Autodesk Fusion 360 part; units mm, degrees
note: some values were not read from the file. Set by a fixed rule: which sketch regions a step uses.
(part 5 of 7)
  line L178 (-125, 205) -> (-105, 195)
  line L179 (-36.1991, -37.2933) -> (-30, -37.2933)
  line L180 (-60.0369, -43.8903) -> (-55.0369, -43.8903)
  line L181 (-55.0369, -43.8903) -> (-55.0369, -37.2933)
  line L182 (-55.0369, -37.2933) -> (-60, -37.2933)
  line L183 (-60, -37.2933) -> (-60, 10)
  line L184 (-60, 10) -> (-55, 10)
  constraint vertical L132
  constraint parallel L131 L133
  constraint parallel L132 L134
  constraint parallel L134 L135
  constraint parallel L134 L137
  constraint parallel L136 L138
  constraint parallel L133 L139
  constraint vertical L140
  constraint parallel L133 L141
  constraint parallel L140 L142
  constraint parallel L142 L143
  constraint parallel L143 L145
  constraint parallel L144 L146
  constraint parallel L139 L147
  constraint parallel L143 L148
  constraint parallel L139 L149
  constraint parallel L143 L150
  constraint parallel L143 L151
  constraint parallel L146 L152
  constraint parallel L151 L153
  constraint parallel L152 L154
  constraint parallel L147 L155
  constraint parallel L151 L156
  constraint parallel L147 L157
  constraint parallel L151 L158
  constraint parallel L151 L159
  constraint parallel L152 L160
  constraint parallel L151 L161
  constraint parallel L160 L162
  constraint parallel L155 L163
  constraint parallel L159 L164
  constraint parallel L163 L165
  constraint parallel L159 L166
  constraint parallel L159 L167
  constraint parallel L159 L169
  constraint parallel L168 L170
  constraint parallel L163 L171
  constraint parallel L167 L172
  constraint parallel L171 L173
  constraint parallel L167 L174
  constraint vertical L175
  constraint parallel L175 L177
  constraint parallel L176 L178
sketch "Sketch89" plane through (0, 116.2145, -31.1396) normal (0, 0.965926, -0.258819) x (-1, 0, 0)
  line L0 (-80, 205) -> (-100, 195)
  line L1 (-100, 195) -> (-100, 200)
  line L2 (-100, 200) -> (-80, 210)
  line L3 (-80, 210) -> (-80, 205)
  line L4 (-105, 170) -> (-105, 165)
  line L5 (-105, 165) -> (-125, 175)
  line L6 (-125, 175) -> (-125, 180)
  line L7 (-125, 180) -> (-105, 170)
  line L8 (-80, 165) -> (-100, 155)
  line L9 (-100, 155) -> (-100, 160)
  line L10 (-100, 160) -> (-80, 170)
  line L11 (-80, 170) -> (-80, 165)
  line L12 (-80, 155) -> (-100, 145)
  line L13 (-100, 145) -> (-100, 150)
  line L14 (-100, 150) -> (-80, 160)
  line L15 (-80, 160) -> (-80, 155)
  line L16 (-105, 180) -> (-105, 175)
  line L17 (-105, 175) -> (-125, 185)
  line L18 (-125, 185) -> (-125, 190)
  line L19 (-125, 190) -> (-105, 180)
  line L20 (-80, 195) -> (-100, 185)
  line L21 (-100, 185) -> (-100, 190)
  line L22 (-100, 190) -> (-80, 200)
  line L23 (-80, 200) -> (-80, 195)
  line L24 (-105, 200) -> (-105, 195)
  line L25 (-105, 195) -> (-125, 205)
  line L26 (-125, 205) -> (-125, 210)
  line L27 (-125, 210) -> (-105, 200)
  line L28 (-105, 160) -> (-105, 155)
  line L29 (-105, 155) -> (-125, 165)
  line L30 (-125, 165) -> (-125, 170)
  line L31 (-125, 170) -> (-105, 160)
  line L32 (-80, 175) -> (-100, 165)
  line L33 (-100, 165) -> (-100, 170)
  line L34 (-100, 170) -> (-80, 180)
  line L35 (-80, 180) -> (-80, 175)
  line L36 (-105, 150) -> (-105, 145)
  line L37 (-105, 145) -> (-125, 155)
  line L38 (-125, 155) -> (-125, 160)
  line L39 (-125, 160) -> (-105, 150)
  line L40 (-105, 190) -> (-105, 185)
  line L41 (-105, 185) -> (-125, 195)
  line L42 (-125, 195) -> (-125, 200)
  line L43 (-125, 200) -> (-105, 190)
  line L44 (-80, 185) -> (-100, 175)
  line L45 (-100, 175) -> (-100, 180)
  line L46 (-100, 180) -> (-80, 190)
  line L47 (-80, 190) -> (-80, 185)
  line L48 (-35.9419, 179.9959) -> (-35.9419, 150.9959)
  line L49 (-35.9419, 150.9959) -> (-72.9419, 150.9959)
  line L50 (-72.9419, 150.9959) -> (-72.9419, 179.9959)
  line L51 (-72.9419, 179.9959) -> (-35.9419, 179.9959)
  line L52 (25, 155) -> (0, 145)
  line L53 (0, 145) -> (0, 150)
  line L54 (0, 150) -> (25, 160)
  line L55 (25, 160) -> (25, 155)
  line L56 (25, 195) -> (0, 185)
  line L57 (0, 185) -> (0, 190)
  line L58 (0, 190) -> (25, 200)
  line L59 (25, 200) -> (25, 195)
  line L60 (-30, 180) -> (-30, 184.9041)
  line L61 (-30, 184.9041) -> (-5, 180)
  line L62 (-5, 180) -> (-5, 175)
  line L63 (-5, 175) -> (-30, 180)
  line L64 (-30, 150) -> (-30, 155)
  line L65 (-30, 155) -> (-5, 150)
  line L66 (-5, 150) -> (-5, 145)
  line L67 (-5, 145) -> (-30, 150)
  line L68 (-5, 190) -> (-5, 184.9041)
  line L69 (-5, 184.9041) -> (-30, 189.9041)
  line L70 (-30, 189.9041) -> (-30, 195)
  line L71 (-30, 195) -> (-5, 190)
  line L72 (25, 185) -> (0, 175)
  line L73 (0, 175) -> (0, 180.1897)
  line L74 (0, 180.1897) -> (25, 190.1897)
  line L75 (25, 190.1897) -> (25, 185)
  line L76 (25, 165) -> (0, 155)
  line L77 (0, 155) -> (0, 160)
  line L78 (0, 160) -> (25, 170)
  line L79 (25, 170) -> (25, 165)
  line L80 (25, 205) -> (0, 195)
  line L81 (0, 195) -> (0, 200)
  line L82 (0, 200) -> (25, 210)
  line L83 (25, 210) -> (25, 205)
  line L84 (-30, 170) -> (-30, 175)
  line L85 (-30, 175) -> (-5, 170)
  line L86 (-5, 170) -> (-5, 165)
  line L87 (-5, 165) -> (-30, 170)
  line L88 (-30, 160) -> (-30, 165.149)
  line L89 (-30, 165.149) -> (-5, 160.149)
  line L90 (-5, 160.149) -> (-5, 155)
  line L91 (-5, 155) -> (-30, 160)
  line L92 (-30, 200) -> (-30, 205)
  line L93 (-30, 205) -> (-5, 200)
  line L94 (-5, 200) -> (-5, 195)
  line L95 (-5, 195) -> (-30, 200)
  line L96 (25, 180.1705) -> (25, 175)
  line L97 (25, 175) -> (0, 165)
  line L98 (0, 165) -> (0, 170)
  line L99 (0, 170) -> (25, 180.1705)
  line L100 (-55, 27.1913) -> (-36.1991, 27.1913)
  line L101 (-36.1991, 27.1913) -> (-36.1991, -37.2933)
  line L102 (-30, -37.2933) -> (-30, -46.5838)
  line L103 (-30, -46.5838) -> (22.741, -46.5838)
  ellipse E0 centre (22.741, -39.3535) end of major axis (22.741, -46.5838) minor radius 7 (22.741, -46.5838) -> (29.741, -39.3535) ccw
  line L104 (29.741, -39.3535) -> (29.741, 209.5755)
  ellipse E1 centre (22.741, 209.5755) end of major axis (22.741, 216.8058) minor radius 7 (29.741, 209.5755) -> (22.741, 216.8058) ccw
  line L105 (22.741, 216.8058) -> (-123.259, 216.8058)
  ellipse E2 centre (-123.259, 209.5755) end of major axis (-123.259, 216.8058) minor radius 7 (-123.259, 216.8058) -> (-130.259, 209.5755) ccw
  line L106 (-130.259, 209.5755) -> (-130.259, -39.3535)
  ellipse E3 centre (-123.259, -39.3535) end of major axis (-123.259, -46.5838) minor radius 7 (-130.259, -39.3535) -> (-123.259, -46.5838) ccw
  line L107 (-123.259, -46.5838) -> (-60.0369, -46.5838)
  line L108 (-60.0369, -46.5838) -> (-60.0369, -43.8903)
  line L109 (-55, 10) -> (-55, 27.1913)
  line L110 (-63.1164, 198.8989) -> (-63.1164, 200.1093)
  line L111 (-63.1164, 200.1093) -> (-65.0274, 200.1093)
  line L112 (-65.0274, 200.1093) -> (-65.0274, 200.872)
  line L113 (-65.0274, 200.872) -> (-62.274, 200.8764)
  line L114 (-62.274, 200.8764) -> (-62.274, 198.4644)
  spline S0 degree 3 poles (-62.274, 198.4644) (-62.4834, 198.3077) (-62.8901, 198.0035) (-63.356, 197.8018) (-63.582, 197.704) knots 0 0 0 0 0.078157 0.151758 0.151758 0.151758 0.151758
  spline S1 degree 3 poles (-63.582, 197.704) (-63.8076, 197.6296) (-64.2571, 197.4815) (-64.7299, 197.4598) (-64.9653, 197.449) knots 0 0 0 0 0.070908 0.141252 0.141252 0.141252 0.141252
  spline S2 degree 3 poles (-64.9653, 197.449) (-65.2744, 197.4647) (-65.8798, 197.4952) (-66.4342, 197.7396) (-66.7056, 197.8592) knots 0 0 0 0 0.091966 0.180141 0.180141 0.180141 0.180141
  spline S3 degree 3 poles (-66.7056, 197.8592) (-66.9503, 198.0107) (-67.4379, 198.3127) (-67.7378, 198.8016) (-67.8872, 199.0452) knots 0 0 0 0 0.085037 0.169503 0.169503 0.169503 0.169503
  spline S4 degree 3 poles (-67.8872, 199.0452) (-68.0036, 199.3151) (-68.2421, 199.8684) (-68.2713, 200.4705) (-68.2863, 200.7789) knots 0 0 0 0 0.087419 0.179189 0.179189 0.179189 0.179189
  spline S5 degree 3 poles (-68.2863, 200.7789) (-68.2704, 201.0885) (-68.239, 201.7016) (-68.0052, 202.2692) (-67.8895, 202.5502) knots 0 0 0 0 0.09226 0.182704 0.182704 0.182704 0.182704
  spline S6 degree 3 poles (-67.8895, 202.5502) (-67.7454, 202.8052) (-67.4631, 203.3049) (-66.9829, 203.6183) (-66.7477, 203.7717) knots 0 0 0 0 0.086466 0.169395 0.169395 0.169395 0.169395
  spline S7 degree 3 poles (-66.7477, 203.7717) (-66.4845, 203.888) (-65.9383, 204.1295) (-65.3412, 204.1567) (-65.0319, 204.1707) knots 0 0 0 0 0.085548 0.177538 0.177538 0.177538 0.177538
  spline S8 degree 3 poles (-65.0319, 204.1707) (-64.8061, 204.1627) (-64.3702, 204.147) (-63.9566, 204.009) (-63.7571, 203.9424) knots 0 0 0 0 0.067359 0.130098 0.130098 0.130098 0.130098
  spline S9 degree 3 poles (-63.7571, 203.9424) (-63.58, 203.862) (-63.2405, 203.7078) (-62.9856, 203.4361) (-62.8637, 203.3061) knots 0 0 0 0 0.057702 0.110632 0.110632 0.110632 0.110632
  spline S10 degree 3 poles (-62.8637, 203.3061) (-62.7607, 203.1533) (-62.5397, 202.8254) (-62.4301, 202.445) (-62.3716, 202.242) knots 0 0 0 0 0.054958 0.117884 0.117884 0.117884 0.117884
  line L115 (-62.3716, 202.242) -> (-63.1475, 202.0292)
  spline S11 degree 3 poles (-63.1475, 202.0292) (-63.1952, 202.1803) (-63.2823, 202.4566) (-63.4397, 202.6995) (-63.5111, 202.8096) knots 0 0 0 0 0.047276 0.086437 0.086437 0.086437 0.086437
  spline S12 degree 3 poles (-63.5111, 202.8096) (-63.5945, 202.9008) (-63.7708, 203.0935) (-64.0072, 203.2052) (-64.1318, 203.264) knots 0 0 0 0 0.036726 0.077589 0.077589 0.077589 0.077589
  spline S13 degree 3 poles (-64.1318, 203.264) (-64.2723, 203.3138) (-64.562, 203.4164) (-64.8692, 203.4285) (-65.0274, 203.4347) knots 0 0 0 0 0.044449 0.091641 0.091641 0.091641 0.091641
  spline S14 degree 3 poles (-65.0274, 203.4347) (-65.2124, 203.4292) (-65.5614, 203.4188) (-65.8919, 203.3075) (-66.0472, 203.2552) knots 0 0 0 0 0.055163 0.104053 0.104053 0.104053 0.104053
  spline S15 degree 3 poles (-66.0472, 203.2552) (-66.1815, 203.1929) (-66.439, 203.0735) (-66.6434, 202.877) (-66.7411, 202.7829) knots 0 0 0 0 0.044061 0.084453 0.084453 0.084453 0.084453
  spline S16 degree 3 poles (-66.7411, 202.7829) (-66.8239, 202.6836) (-66.988, 202.4867) (-67.0971, 202.2549) (-67.1512, 202.14) knots 0 0 0 0 0.038631 0.076535 0.076535 0.076535 0.076535
  spline S17 degree 3 poles (-67.1512, 202.14) (-67.2236, 201.9325) (-67.3714, 201.509) (-67.39, 201.0607) (-67.3995, 200.8321) knots 0 0 0 0 0.06555 0.133782 0.133782 0.133782 0.133782
  spline S18 degree 3 poles (-67.3995, 200.8321) (-67.3911, 200.5625) (-67.3753, 200.0597) (-67.1874, 199.5938) (-67.1002, 199.3778) knots 0 0 0 0 0.080159 0.149513 0.149513 0.149513 0.149513
  spline S19 degree 3 poles (-67.1002, 199.3778) (-66.9899, 199.1956) (-66.7709, 198.8342) (-66.4087, 198.6166) (-66.229, 198.5087) knots 0 0 0 0 0.06285 0.12472 0.12472 0.12472 0.12472
  spline S20 degree 3 poles (-66.229, 198.5087) (-66.0352, 198.426) (-65.6469, 198.2601) (-65.2253, 198.2367) (-65.0141, 198.225) knots 0 0 0 0 0.062693 0.125611 0.125611 0.125611 0.125611
  spline S21 degree 3 poles (-65.0141, 198.225) (-64.8284, 198.2342) (-64.4544, 198.2527) (-64.1012, 198.3773) (-63.9234, 198.44) knots 0 0 0 0 0.055462 0.111696 0.111696 0.111696 0.111696
  spline S22 degree 3 poles (-63.9234, 198.44) (-63.7635, 198.5072) (-63.4759, 198.6281) (-63.227, 198.8156) (-63.1164, 198.8989) knots 0 0 0 0 0.051788 0.093147 0.093147 0.093147 0.093147
  spline S23 degree 3 poles (-54.9382, 198.3003) (-54.9002, 198.2836) (-54.8136, 198.2455) (-54.7187, 198.2437) (-54.6656, 198.2427) knots 0 0 0 0 0.012364 0.028114 0.028114 0.028114 0.028114
  spline S24 degree 3 poles (-54.6656, 198.2427) (-54.6141, 198.2445) (-54.4969, 198.2487) (-54.3806, 198.2647) (-54.3153, 198.2737) knots 0 0 0 0 0.015427 0.035185 0.035185 0.035185 0.035185
  line L116 (-54.3153, 198.2737) -> (-54.2, 197.5688)
  spline S25 degree 3 poles (-54.2, 197.5688) (-54.3061, 197.5481) (-54.5053, 197.5093) (-54.7082, 197.5015) (-54.803, 197.4978) knots 0 0 0 0 0.032364 0.060796 0.060796 0.060796 0.060796
  spline S26 degree 3 poles (-54.803, 197.4978) (-54.9335, 197.5003) (-55.1673, 197.5048) (-55.3821, 197.5953) (-55.4769, 197.6353) knots 0 0 0 0 0.038727 0.069335 0.069335 0.069335 0.069335
  spline S27 degree 3 poles (-55.4769, 197.6353) (-55.5503, 197.6834) (-55.6922, 197.7765) (-55.7742, 197.9249) (-55.8139, 197.9966) knots 0 0 0 0 0.025865 0.050076 0.050076 0.050076 0.050076
  spline S28 degree 3 poles (-55.8139, 197.9966) (-55.842, 198.112) (-55.917, 198.4208) (-55.9136, 198.7393) (-55.9115, 198.9388) knots 0 0 0 0 0.035512 0.095031 0.095031 0.095031 0.095031
  line L117 (-55.9115, 198.9388) -> (-55.9115, 201.6479)
  line L118 (-55.9115, 201.6479) -> (-56.4967, 201.6479)
  line L119 (-56.4967, 201.6479) -> (-56.4967, 202.2686)
  line L120 (-56.4967, 202.2686) -> (-55.9115, 202.2686)
  line L121 (-55.9115, 202.2686) -> (-55.9115, 203.4347)
  line L122 (-55.9115, 203.4347) -> (-55.1178, 203.9136)
  line L123 (-55.1178, 203.9136) -> (-55.1178, 202.2686)
  line L124 (-55.1178, 202.2686) -> (-54.3153, 202.2686)
  line L125 (-54.3153, 202.2686) -> (-54.3153, 201.6479)
  line L126 (-54.3153, 201.6479) -> (-55.1178, 201.6479)
  line L127 (-55.1178, 201.6479) -> (-55.1178, 198.8945)
  spline S29 degree 3 poles (-55.1178, 198.8945) (-55.119, 198.8004) (-55.1208, 198.6523) (-55.0878, 198.5082) (-55.0757, 198.4555) knots 0 0 0 0 0.028064 0.044226 0.044226 0.044226 0.044226
  spline S30 degree 3 poles (-55.0757, 198.4555) (-55.0592, 198.4246) (-55.0259, 198.3618) (-54.9677, 198.321) (-54.9382, 198.3003) knots 0 0 0 0 0.010363 0.020994 0.020994 0.020994 0.020994
  line L128 (-47.6823, 204.0599) -> (-47.6823, 203.1421)
  line L129 (-47.6823, 203.1421) -> (-48.4804, 203.1421)
  line L130 (-48.4804, 203.1421) -> (-48.4804, 204.0599)
  line L131 (-48.4804, 204.0599) -> (-47.6823, 204.0599)
  spline S31 degree 3 poles (-45.3434, 188.1557) (-45.3053, 188.139) (-45.2188, 188.1009) (-45.1239, 188.0991) (-45.0707, 188.0981) knots 0 0 0 0 0.012364 0.028115 0.028115 0.028115 0.028115
  spline S32 degree 3 poles (-45.0707, 188.0981) (-45.0193, 188.0999) (-44.902, 188.1041) (-44.7858, 188.1201) (-44.7205, 188.1291) knots 0 0 0 0 0.015427 0.035184 0.035184 0.035184 0.035184
  line L132 (-44.7205, 188.1291) -> (-44.6052, 187.4241)
  spline S33 degree 3 poles (-44.6052, 187.4241) (-44.7113, 187.4035) (-44.9105, 187.3647) (-45.1133, 187.3569) (-45.2082, 187.3532) knots 0 0 0 0 0.032364 0.060796 0.060796 0.060796 0.060796
  spline S34 degree 3 poles (-45.2082, 187.3532) (-45.3387, 187.3557) (-45.5725, 187.3602) (-45.7873, 187.4507) (-45.8821, 187.4907) knots 0 0 0 0 0.038727 0.069335 0.069335 0.069335 0.069335
  spline S35 degree 3 poles (-45.8821, 187.4907) (-45.9554, 187.5388) (-46.0974, 187.6319) (-46.1794, 187.7803) (-46.2191, 187.852) knots 0 0 0 0 0.025865 0.050076 0.050076 0.050076 0.050076
  spline S36 degree 3 poles (-46.2191, 187.852) (-46.2471, 187.9674) (-46.3222, 188.2761) (-46.3188, 188.5947) (-46.3166, 188.7942) knots 0 0 0 0 0.035512 0.095031 0.095031 0.095031 0.095031
  line L133 (-46.3166, 188.7942) -> (-46.3166, 191.5033)
  line L134 (-46.3166, 191.5033) -> (-46.9019, 191.5033)
  line L135 (-46.9019, 191.5033) -> (-46.9019, 192.124)
  line L136 (-46.9019, 192.124) -> (-46.3166, 192.124)
  line L137 (-46.3166, 192.124) -> (-46.3166, 193.2901)
  line L138 (-46.3166, 193.2901) -> (-45.523, 193.769)
  line L139 (-45.523, 193.769) -> (-45.523, 192.124)
  line L140 (-45.523, 192.124) -> (-44.7205, 192.124)
  line L141 (-44.7205, 192.124) -> (-44.7205, 191.5033)
  line L142 (-44.7205, 191.5033) -> (-45.523, 191.5033)
  line L143 (-45.523, 191.5033) -> (-45.523, 188.7499)
  spline S37 degree 3 poles (-45.523, 188.7499) (-45.5242, 188.6558) (-45.526, 188.5076) (-45.4929, 188.3636) (-45.4809, 188.3109) knots 0 0 0 0 0.028064 0.044226 0.044226 0.044226 0.044226
  spline S38 degree 3 poles (-45.4809, 188.3109) (-45.4644, 188.2799) (-45.4311, 188.2172) (-45.3729, 188.1764) (-45.3434, 188.1557) knots 0 0 0 0 0.010363 0.020994 0.020994 0.020994 0.020994
  line L144 (-67.1956, 190.3017) -> (-67.1956, 187.4153)
  line L145 (-67.1956, 187.4153) -> (-68.0557, 187.4153)
  line L146 (-68.0557, 187.4153) -> (-68.0557, 193.9153)
  line L147 (-68.0557, 193.9153) -> (-65.1737, 193.9153)
  spline S39 degree 3 poles (-65.1737, 193.9153) (-64.917, 193.9133) (-64.4685, 193.9099) (-64.0369, 193.791) (-63.8525, 193.7401) knots 0 0 0 0 0.076609 0.133783 0.133783 0.133783 0.133783
  spline S40 degree 3 poles (-63.8525, 193.7401) (-63.7085, 193.6693) (-63.4151, 193.5248) (-63.226, 193.2577) (-63.1297, 193.1216) knots 0 0 0 0 0.047344 0.096479 0.096479 0.096479 0.096479
  spline S41 degree 3 poles (-63.1297, 193.1216) (-63.0509, 192.9692) (-62.8917, 192.6617) (-62.8702, 192.3161) (-62.8593, 192.1417) knots 0 0 0 0 0.050884 0.102649 0.102649 0.102649 0.102649
  spline S42 degree 3 poles (-62.8593, 192.1417) (-62.8767, 191.9216) (-62.911, 191.4883) (-63.1765, 191.1447) (-63.3071, 190.9756) knots 0 0 0 0 0.064712 0.127351 0.127351 0.127351 0.127351
  spline S43 degree 3 poles (-63.3071, 190.9756) (-63.4898, 190.8304) (-63.8954, 190.5079) (-64.4084, 190.4206) (-64.6905, 190.3726) knots 0 0 0 0 0.068929 0.153084 0.153084 0.153084 0.153084
  spline S44 degree 3 poles (-64.6905, 190.3726) (-64.588, 190.322) (-64.4042, 190.2312) (-64.243, 190.1049) (-64.1717, 190.049) knots 0 0 0 0 0.034174 0.061288 0.061288 0.061288 0.061288
  spline S45 degree 3 poles (-64.1717, 190.049) (-64.0453, 189.9227) (-63.7798, 189.6574) (-63.5685, 189.347) (-63.4578, 189.1844) knots 0 0 0 0 0.053478 0.112342 0.112342 0.112342 0.112342
  line L148 (-63.4578, 189.1844) -> (-62.3272, 187.4153)
  line L149 (-62.3272, 187.4153) -> (-63.4091, 187.4153)
  line L150 (-63.4091, 187.4153) -> (-64.2692, 188.7676)
  spline S46 degree 3 poles (-64.2692, 188.7676) (-64.3816, 188.9413) (-64.5791, 189.2464) (-64.7964, 189.5377) (-64.89, 189.6632) knots 0 0 0 0 0.06204 0.108997 0.108997 0.108997 0.108997
  spline S47 degree 3 poles (-64.89, 189.6632) (-64.9633, 189.7549) (-65.0926, 189.9165) (-65.256, 190.043) (-65.3267, 190.0977) knots 0 0 0 0 0.035073 0.061797 0.061797 0.061797 0.061797
  spline S48 degree 3 poles (-65.3267, 190.0977) (-65.3903, 190.1357) (-65.514, 190.2097) (-65.652, 190.2507) (-65.7191, 190.2707) knots 0 0 0 0 0.022121 0.04303 0.04303 0.04303 0.04303
  spline S49 degree 3 poles (-65.7191, 190.2707) (-65.7833, 190.2796) (-65.942, 190.3018) (-66.1024, 190.3018) (-66.198, 190.3017) knots 0 0 0 0 0.019427 0.048036 0.048036 0.048036 0.048036
  line L151 (-66.198, 190.3017) -> (-67.1956, 190.3017)
  spline S50 degree 3 poles (-54.5192, 187.3089) (-54.7824, 187.3382) (-55.3103, 187.3972) (-55.6546, 187.8019) (-55.8272, 188.005) knots 0 0 0 0 0.076386 0.153256 0.153256 0.153256 0.153256
  line L152 (-55.8272, 188.005) -> (-55.8272, 187.4153)
  line L153 (-55.8272, 187.4153) -> (-56.5677, 187.4153)
  line L154 (-56.5677, 187.4153) -> (-56.5677, 193.9153)
  line L155 (-56.5677, 193.9153) -> (-55.7696, 193.9153)
  line L156 (-55.7696, 193.9153) -> (-55.7696, 191.5964)
  spline S51 degree 3 poles (-55.7696, 191.5964) (-55.5907, 191.7813) (-55.2364, 192.1477) (-54.7301, 192.203) (-54.4793, 192.2304) knots 0 0 0 0 0.074638 0.14787 0.14787 0.14787 0.14787
  spline S52 degree 3 poles (-54.4793, 192.2304) (-54.3368, 192.2233) (-54.0532, 192.2091) (-53.7885, 192.1064) (-53.6569, 192.0553) knots 0 0 0 0 0.042514 0.084577 0.084577 0.084577 0.084577
  spline S53 degree 3 poles (-53.6569, 192.0553) (-53.5338, 191.9917) (-53.2911, 191.8663) (-53.1085, 191.6633) (-53.0184, 191.5631) knots 0 0 0 0 0.041157 0.081209 0.081209 0.081209 0.081209
  spline S54 degree 3 poles (-53.0184, 191.5631) (-52.9386, 191.4493) (-52.7726, 191.2126) (-52.6761, 190.9399) (-52.626, 190.7983) knots 0 0 0 0 0.041496 0.086317 0.086317 0.086317 0.086317
  spline S55 degree 3 poles (-52.626, 190.7983) (-52.5846, 190.6447) (-52.5001, 190.3311) (-52.4895, 190.0063) (-52.4841, 189.8406) knots 0 0 0 0 0.04754 0.097104 0.097104 0.097104 0.097104
  spline S56 degree 3 poles (-52.4841, 189.8406) (-52.4995, 189.4713) (-52.528, 188.7899) (-52.9084, 188.2272) (-53.0827, 187.9695) knots 0 0 0 0 0.108337 0.199906 0.199906 0.199906 0.199906
  spline S57 degree 3 poles (-53.0827, 187.9695) (-53.2896, 187.7768) (-53.6964, 187.3982) (-54.2482, 187.3383) (-54.5192, 187.3089) knots 0 0 0 0 0.082403 0.16195 0.16195 0.16195 0.16195
  spline S58 degree 3 poles (-49.6021, 187.3089) (-49.9123, 187.3316) (-50.5128, 187.3757) (-50.9764, 187.758) (-51.2005, 187.9429) knots 0 0 0 0 0.090792 0.175782 0.175782 0.175782 0.175782
  spline S59 degree 3 poles (-51.2005, 187.9429) (-51.378, 188.192) (-51.7656, 188.7359) (-51.7945, 189.4063) (-51.8102, 189.7696) knots 0 0 0 0 0.089871 0.196272 0.196272 0.196272 0.196272
  spline S60 degree 3 poles (-51.8102, 189.7696) (-51.792, 190.166) (-51.7585, 190.8949) (-51.2947, 191.4527) (-51.083, 191.7072) knots 0 0 0 0 0.115281 0.212035 0.212035 0.212035 0.212035
  spline S61 degree 3 poles (-51.083, 191.7072) (-50.8662, 191.8598) (-50.422, 192.1723) (-49.8797, 192.2108) (-49.6021, 192.2304) knots 0 0 0 0 0.077985 0.159734 0.159734 0.159734 0.159734
  spline S62 degree 3 poles (-49.6021, 192.2304) (-49.296, 192.2068) (-48.6994, 192.1607) (-48.239, 191.7797) (-48.0148, 191.5942) knots 0 0 0 0 0.089656 0.174785 0.174785 0.174785 0.174785
  spline S63 degree 3 poles (-48.0148, 191.5942) (-47.8353, 191.3509) (-47.4509, 190.8303) (-47.4167, 190.1817) (-47.3985, 189.8362) knots 0 0 0 0 0.08875 0.189968 0.189968 0.189968 0.189968
  spline S64 degree 3 poles (-47.3985, 189.8362) (-47.4038, 189.5619) (-47.4134, 189.0687) (-47.5919, 188.61) (-47.6712, 188.4062) knots 0 0 0 0 0.08148 0.146573 0.146573 0.146573 0.146573
  spline S65 degree 3 poles (-47.6712, 188.4062) (-47.7727, 188.2421) (-47.9764, 187.9128) (-48.3017, 187.7025) (-48.4648, 187.5971) knots 0 0 0 0 0.057116 0.114612 0.114612 0.114612 0.114612
  spline S66 degree 3 poles (-48.4648, 187.5971) (-48.6434, 187.513) (-49.0037, 187.3434) (-49.4015, 187.3204) (-49.6021, 187.3089) knots 0 0 0 0 0.058612 0.118296 0.118296 0.118296 0.118296
  spline S67 degree 3 poles (-59.7024, 187.3089) (-60.0126, 187.3316) (-60.6131, 187.3757) (-61.0766, 187.758) (-61.3008, 187.9429) knots 0 0 0 0 0.090792 0.175782 0.175782 0.175782 0.175782
  spline S68 degree 3 poles (-61.3008, 187.9429) (-61.4783, 188.192) (-61.8659, 188.7359) (-61.8948, 189.4063) (-61.9104, 189.7696) knots 0 0 0 0 0.089871 0.196272 0.196272 0.196272 0.196272
  spline S69 degree 3 poles (-61.9104, 189.7696) (-61.8922, 190.166) (-61.8588, 190.8949) (-61.3949, 191.4527) (-61.1833, 191.7072) knots 0 0 0 0 0.115281 0.212035 0.212035 0.212035 0.212035
  spline S70 degree 3 poles (-61.1833, 191.7072) (-60.9664, 191.8598) (-60.5223, 192.1723) (-59.9799, 192.2108) (-59.7024, 192.2304) knots 0 0 0 0 0.077985 0.159734 0.159734 0.159734 0.159734
  spline S71 degree 3 poles (-59.7024, 192.2304) (-59.3963, 192.2068) (-58.7996, 192.1607) (-58.3393, 191.7797) (-58.1151, 191.5942) knots 0 0 0 0 0.089656 0.174785 0.174785 0.174785 0.174785
  spline S72 degree 3 poles (-58.1151, 191.5942) (-57.9355, 191.3509) (-57.5512, 190.8303) (-57.517, 190.1817) (-57.4988, 189.8362) knots 0 0 0 0 0.08875 0.189968 0.189968 0.189968 0.189968
  spline S73 degree 3 poles (-57.4988, 189.8362) (-57.5041, 189.5619) (-57.5137, 189.0687) (-57.6922, 188.61) (-57.7715, 188.4062) knots 0 0 0 0 0.08148 0.146573 0.146573 0.146573 0.146573
  spline S74 degree 3 poles (-57.7715, 188.4062) (-57.873, 188.2421) (-58.0767, 187.9128) (-58.4019, 187.7025) (-58.5651, 187.5971) knots 0 0 0 0 0.057116 0.114612 0.114612 0.114612 0.114612
  spline S75 degree 3 poles (-58.5651, 187.5971) (-58.7437, 187.513) (-59.104, 187.3434) (-59.5017, 187.3204) (-59.7024, 187.3089) knots 0 0 0 0 0.058612 0.118295 0.118295 0.118295 0.118295
  line L157 (-45.6693, 200.1315) -> (-45.6693, 197.5599)
  line L158 (-45.6693, 197.5599) -> (-46.4674, 197.5599)
  line L159 (-46.4674, 197.5599) -> (-46.4674, 202.2686)
  line L160 (-46.4674, 202.2686) -> (-45.7491, 202.2686)
  line L161 (-45.7491, 202.2686) -> (-45.7491, 201.5991)
  spline S76 degree 3 poles (-45.7491, 201.5991) (-45.5547, 201.8254) (-45.16, 202.2847) (-44.5566, 202.3446) (-44.2505, 202.375) knots 0 0 0 0 0.086062 0.174671 0.174671 0.174671 0.174671
  spline S77 degree 3 poles (-44.2505, 202.375) (-44.1129, 202.3693) (-43.8442, 202.3581) (-43.5913, 202.2667) (-43.4679, 202.2221) knots 0 0 0 0 0.041025 0.080156 0.080156 0.080156 0.080156
  spline S78 degree 3 poles (-43.4679, 202.2221) (-43.3586, 202.1701) (-43.153, 202.0722) (-43.0036, 201.901) (-42.9336, 201.8208) knots 0 0 0 0 0.035864 0.067451 0.067451 0.067451 0.067451
  spline S79 degree 3 poles (-42.9336, 201.8208) (-42.8786, 201.7323) (-42.7645, 201.5491) (-42.7123, 201.3395) (-42.6853, 201.2311) knots 0 0 0 0 0.031061 0.064335 0.064335 0.064335 0.064335
  spline S80 degree 3 poles (-42.6853, 201.2311) (-42.6725, 201.1296) (-42.6401, 200.8721) (-42.6407, 200.6125) (-42.641, 200.4552) knots 0 0 0 0 0.030663 0.077786 0.077786 0.077786 0.077786
  line L162 (-42.641, 200.4552) -> (-42.641, 197.5599)
  line L163 (-42.641, 197.5599) -> (-43.4391, 197.5599)
  line L164 (-43.4391, 197.5599) -> (-43.4391, 200.4241)
  spline S81 degree 3 poles (-43.4391, 200.4241) (-43.4399, 200.5672) (-43.4412, 200.8145) (-43.5052, 201.053) (-43.5322, 201.1535) knots 0 0 0 0 0.042684 0.073794 0.073794 0.073794 0.073794
  spline S82 degree 3 poles (-43.5322, 201.1535) (-43.57, 201.2304) (-43.6469, 201.3872) (-43.7898, 201.4879) (-43.8625, 201.5393) knots 0 0 0 0 0.025274 0.051516 0.051516 0.051516 0.051516
  spline S83 degree 3 poles (-43.8625, 201.5393) (-43.9468, 201.5813) (-44.122, 201.6685) (-44.3176, 201.6783) (-44.419, 201.6834) knots 0 0 0 0 0.027946 0.058036 0.058036 0.058036 0.058036
  spline S84 degree 3 poles (-44.419, 201.6834) (-44.5825, 201.6704) (-44.9063, 201.6448) (-45.169, 201.4541) (-45.2991, 201.3597) knots 0 0 0 0 0.048182 0.095412 0.095412 0.095412 0.095412
  spline S85 degree 3 poles (-45.2991, 201.3597) (-45.4063, 201.2084) (-45.6641, 200.8447) (-45.6674, 200.3945) (-45.6693, 200.1315) knots 0 0 0 0 0.054493 0.130984 0.130984 0.130984 0.130984
  line L165 (-47.6823, 202.2686) -> (-47.6823, 197.5599)
  line L166 (-47.6823, 197.5599) -> (-48.4804, 197.5599)
  line L167 (-48.4804, 197.5599) -> (-48.4804, 202.2686)
  line L168 (-48.4804, 202.2686) -> (-47.6823, 202.2686)
  line L169 (-52.7368, 200.1359) -> (-52.7368, 197.5599)
  line L170 (-52.7368, 197.5599) -> (-53.5349, 197.5599)
  line L171 (-53.5349, 197.5599) -> (-53.5349, 204.0599)
  line L172 (-53.5349, 204.0599) -> (-52.7368, 204.0599)
  line L173 (-52.7368, 204.0599) -> (-52.7368, 201.7277)
  spline S86 degree 3 poles (-52.7368, 201.7277) (-52.5386, 201.9165) (-52.1426, 202.2936) (-51.5986, 202.3479) (-51.3269, 202.375) knots 0 0 0 0 0.079682 0.15916 0.15916 0.15916 0.15916
  spline S87 degree 3 poles (-51.3269, 202.375) (-51.1615, 202.3682) (-50.8456, 202.355) (-50.556, 202.229) (-50.4179, 202.1689) knots 0 0 0 0 0.049154 0.09392 0.09392 0.09392 0.09392
  spline S88 degree 3 poles (-50.4179, 202.1689) (-50.2992, 202.0951) (-50.0674, 201.9511) (-49.932, 201.7145) (-49.8659, 201.5991) knots 0 0 0 0 0.041202 0.080448 0.080448 0.080448 0.080448
  spline S89 degree 3 poles (-49.8659, 201.5991) (-49.8177, 201.4517) (-49.7057, 201.1097) (-49.7018, 200.7491) (-49.6997, 200.5439) knots 0 0 0 0 0.046272 0.107379 0.107379 0.107379 0.107379
  line L174 (-49.6997, 200.5439) -> (-49.6997, 197.5599)
  line L175 (-49.6997, 197.5599) -> (-50.4977, 197.5599)
  line L176 (-50.4977, 197.5599) -> (-50.4977, 200.5439)
  spline S90 degree 3 poles (-50.4977, 200.5439) (-50.5019, 200.7219) (-50.5093, 201.038) (-50.6818, 201.3005) (-50.7571, 201.4151) knots 0 0 0 0 0.052115 0.092521 0.092521 0.092521 0.092521
  spline S91 degree 3 poles (-50.7571, 201.4151) (-50.8571, 201.4946) (-51.0711, 201.6645) (-51.345, 201.6797) (-51.4909, 201.6878) knots 0 0 0 0 0.037401 0.080016 0.080016 0.080016 0.080016
  spline S92 degree 3 poles (-51.4909, 201.6878) (-51.6077, 201.6799) (-51.8427, 201.6642) (-52.0526, 201.5575) (-52.1582, 201.5038) knots 0 0 0 0 0.034724 0.069859 0.069859 0.069859 0.069859
  spline S93 degree 3 poles (-52.1582, 201.5038) (-52.2546, 201.4379) (-52.4442, 201.3081) (-52.5512, 201.1049) (-52.6038, 201.005) knots 0 0 0 0 0.034441 0.067793 0.067793 0.067793 0.067793
  spline S94 degree 3 poles (-52.6038, 201.005) (-52.6425, 200.881) (-52.7305, 200.5985) (-52.7346, 200.3022) (-52.7368, 200.1359) knots 0 0 0 0 0.038771 0.08832 0.08832 0.08832 0.08832
  spline S95 degree 3 poles (-59.126, 198.1097) (-58.9869, 198.1179) (-58.718, 198.1338) (-58.4878, 198.273) (-58.3767, 198.3402) knots 0 0 0 0 0.041087 0.079456 0.079456 0.079456 0.079456
  spline S96 degree 3 poles (-58.3767, 198.3402) (-58.2764, 198.4349) (-58.0569, 198.6421) (-57.9452, 198.9234) (-57.8845, 199.0763) knots 0 0 0 0 0.040863 0.089495 0.089495 0.089495 0.089495
  line L177 (-57.8845, 199.0763) -> (-57.0598, 198.9743)
  spline S97 degree 3 poles (-57.0598, 198.9743) (-57.1356, 198.7493) (-57.2822, 198.3139) (-57.6195, 198.0028) (-57.7825, 197.8525) knots 0 0 0 0 0.069951 0.135368 0.135368 0.135368 0.135368
  spline S98 degree 3 poles (-57.7825, 197.8525) (-57.9777, 197.7362) (-58.3921, 197.4894) (-58.875, 197.4659) (-59.1304, 197.4535) knots 0 0 0 0 0.06712 0.142493 0.142493 0.142493 0.142493
  spline S99 degree 3 poles (-59.1304, 197.4535) (-59.4518, 197.4748) (-60.0664, 197.5155) (-60.5419, 197.9043) (-60.7687, 198.0897) knots 0 0 0 0 0.093968 0.179695 0.179695 0.179695 0.179695
  spline S100 degree 3 poles (-60.7687, 198.0897) (-60.945, 198.3356) (-61.3258, 198.8668) (-61.3571, 199.5223) (-61.3739, 199.8744) knots 0 0 0 0 0.088891 0.192041 0.192041 0.192041 0.192041
  spline S101 degree 3 poles (-61.3739, 199.8744) (-61.3573, 200.2381) (-61.3265, 200.9133) (-60.9403, 201.4645) (-60.7621, 201.7188) knots 0 0 0 0 0.106628 0.197922 0.197922 0.197922 0.197922
  spline S102 degree 3 poles (-60.7621, 201.7188) (-60.5393, 201.9102) (-60.0829, 202.3022) (-59.4822, 202.3504) (-59.1748, 202.375) knots 0 0 0 0 0.085796 0.175759 0.175759 0.175759 0.175759
  spline S103 degree 3 poles (-59.1748, 202.375) (-58.8765, 202.3505) (-58.292, 202.3025) (-57.8488, 201.9196) (-57.6318, 201.7321) knots 0 0 0 0 0.087287 0.171058 0.171058 0.171058 0.171058
  spline S104 degree 3 poles (-57.6318, 201.7321) (-57.4575, 201.4828) (-57.0794, 200.9419) (-57.0494, 200.28) (-57.0332, 199.9231) knots 0 0 0 0 0.089451 0.194057 0.194057 0.194057 0.194057
  spline S105 degree 3 poles (-57.0332, 199.9231) (-57.0335, 199.8936) (-57.0342, 199.8226) (-57.0364, 199.7517) (-57.0377, 199.7103) knots 0 0 0 0 0.008868 0.021288 0.021288 0.021288 0.021288
  line L178 (-57.0377, 199.7103) -> (-60.5493, 199.7103)
  spline S106 degree 3 poles (-60.5493, 199.7103) (-60.5262, 199.4739) (-60.4836, 199.0377) (-60.2276, 198.684) (-60.1103, 198.522) knots 0 0 0 0 0.069761 0.128713 0.128713 0.128713 0.128713
  spline S107 degree 3 poles (-60.1103, 198.522) (-59.9697, 198.4018) (-59.686, 198.159) (-59.3138, 198.1262) (-59.126, 198.1097) knots 0 0 0 0 0.054058 0.109125 0.109125 0.109125 0.109125
  line L179 (-125, 135) -> (25, 135)
  line L180 (25, 135) -> (25, 130)
  line L181 (25, 130) -> (-125, 130)
  line L182 (-125, 130) -> (-125, 135)
  line L183 (-36.1991, -37.2933) -> (-30, -37.2933)
  line L184 (-60.0369, -43.8903) -> (-55.0369, -43.8903)
  line L185 (-55.0369, -43.8903) -> (-55.0369, -37.2933)
  line L186 (-55.0369, -37.2933) -> (-60, -37.2933)
  line L187 (-60, -37.2933) -> (-60, 10)
  line L188 (-60, 10) -> (-55, 10)
  constraint horizontal L179
  constraint vertical L180
  constraint horizontal L181
  constraint vertical L182
sketch "Sketch90" plane through (0, 116.2145, -31.1396) normal (0, 0.965926, -0.258819) x (-1, 0, 0)
  line L0 (25, 135) -> (25, 130)
  line L1 (25, 130) -> (-125, 130)
  line L2 (-125, 130) -> (-125, 135)
  line L3 (-125, 135) -> (25, 135)
  line L4 (-80, 205) -> (-100, 195)
  line L5 (-100, 195) -> (-100, 200)
  line L6 (-100, 200) -> (-80, 210)
  line L7 (-80, 210) -> (-80, 205)
  line L8 (-105, 170) -> (-105, 165)
  line L9 (-105, 165) -> (-125, 175)
  line L10 (-125, 175) -> (-125, 180)
  line L11 (-125, 180) -> (-105, 170)
  line L12 (-80, 165) -> (-100, 155)
  line L13 (-100, 155) -> (-100, 160)
  line L14 (-100, 160) -> (-80, 170)
  line L15 (-80, 170) -> (-80, 165)
  line L16 (-80, 155) -> (-100, 145)
  line L17 (-100, 145) -> (-100, 150)
  line L18 (-100, 150) -> (-80, 160)
  line L19 (-80, 160) -> (-80, 155)
  line L20 (-105, 180) -> (-105, 175)
  line L21 (-105, 175) -> (-125, 185)
  line L22 (-125, 185) -> (-125, 190)
  line L23 (-125, 190) -> (-105, 180)
  line L24 (-80, 195) -> (-100, 185)
  line L25 (-100, 185) -> (-100, 190)
  line L26 (-100, 190) -> (-80, 200)
  line L27 (-80, 200) -> (-80, 195)
  line L28 (-105, 200) -> (-105, 195)
  line L29 (-105, 195) -> (-125, 205)
  line L30 (-125, 205) -> (-125, 210)
  line L31 (-125, 210) -> (-105, 200)
  line L32 (-105, 160) -> (-105, 155)
  line L33 (-105, 155) -> (-125, 165)
  line L34 (-125, 165) -> (-125, 170)
  line L35 (-125, 170) -> (-105, 160)
  line L36 (-80, 175) -> (-100, 165)
  line L37 (-100, 165) -> (-100, 170)
  line L38 (-100, 170) -> (-80, 180)
  line L39 (-80, 180) -> (-80, 175)
  line L40 (-105, 150) -> (-105, 145)
  line L41 (-105, 145) -> (-125, 155)
  line L42 (-125, 155) -> (-125, 160)
  line L43 (-125, 160) -> (-105, 150)
  line L44 (-105, 190) -> (-105, 185)
  line L45 (-105, 185) -> (-125, 195)
  line L46 (-125, 195) -> (-125, 200)
  line L47 (-125, 200) -> (-105, 190)
  line L48 (-80, 185) -> (-100, 175)
  line L49 (-100, 175) -> (-100, 180)
  line L50 (-100, 180) -> (-80, 190)
  line L51 (-80, 190) -> (-80, 185)
  line L52 (-35.9419, 179.9959) -> (-35.9419, 150.9959)
  line L53 (-35.9419, 150.9959) -> (-72.9419, 150.9959)
  line L54 (-72.9419, 150.9959) -> (-72.9419, 179.9959)
  line L55 (-72.9419, 179.9959) -> (-35.9419, 179.9959)
  line L56 (25, 155) -> (0, 145)
  line L57 (0, 145) -> (0, 150)
  line L58 (0, 150) -> (25, 160)
  line L59 (25, 160) -> (25, 155)
  line L60 (25, 195) -> (0, 185)
  line L61 (0, 185) -> (0, 190)
  line L62 (0, 190) -> (25, 200)
  line L63 (25, 200) -> (25, 195)
  line L64 (-30, 180) -> (-30, 184.9041)
  line L65 (-30, 184.9041) -> (-5, 180)
  line L66 (-5, 180) -> (-5, 175)
  line L67 (-5, 175) -> (-30, 180)
  line L68 (-30, 150) -> (-30, 155)
  line L69 (-30, 155) -> (-5, 150)
  line L70 (-5, 150) -> (-5, 145)
  line L71 (-5, 145) -> (-30, 150)
  line L72 (-5, 190) -> (-5, 184.9041)
  line L73 (-5, 184.9041) -> (-30, 189.9041)
  line L74 (-30, 189.9041) -> (-30, 195)
  line L75 (-30, 195) -> (-5, 190)
  line L76 (25, 185) -> (0, 175)
  line L77 (0, 175) -> (0, 180.1897)
  line L78 (0, 180.1897) -> (25, 190.1897)
  line L79 (25, 190.1897) -> (25, 185)
  line L80 (25, 165) -> (0, 155)
  line L81 (0, 155) -> (0, 160)
  line L82 (0, 160) -> (25, 170)
  line L83 (25, 170) -> (25, 165)
  line L84 (25, 205) -> (0, 195)
  line L85 (0, 195) -> (0, 200)
  line L86 (0, 200) -> (25, 210)
  line L87 (25, 210) -> (25, 205)
  line L88 (-30, 170) -> (-30, 175)
  line L89 (-30, 175) -> (-5, 170)
  line L90 (-5, 170) -> (-5, 165)
  line L91 (-5, 165) -> (-30, 170)
  line L92 (-30, 160) -> (-30, 165.149)
  line L93 (-30, 165.149) -> (-5, 160.149)
  line L94 (-5, 160.149) -> (-5, 155)
  line L95 (-5, 155) -> (-30, 160)
  line L96 (-30, 200) -> (-30, 205)
  line L97 (-30, 205) -> (-5, 200)
  line L98 (-5, 200) -> (-5, 195)
  line L99 (-5, 195) -> (-30, 200)
  line L100 (25, 180.1705) -> (25, 175)
  line L101 (25, 175) -> (0, 165)
  line L102 (0, 165) -> (0, 170)
  line L103 (0, 170) -> (25, 180.1705)
  line L104 (-55, 27.1913) -> (-36.1991, 27.1913)
  line L105 (-36.1991, 27.1913) -> (-36.1991, -37.2933)
  line L106 (-30, -37.2933) -> (-30, -46.5838)
  line L107 (-30, -46.5838) -> (22.741, -46.5838)
  ellipse E0 centre (22.741, -39.3535) end of major axis (22.741, -46.5838) minor radius 7 (22.741, -46.5838) -> (29.741, -39.3535) ccw
  line L108 (29.741, -39.3535) -> (29.741, 209.5755)
  ellipse E1 centre (22.741, 209.5755) end of major axis (22.741, 216.8058) minor radius 7 (29.741, 209.5755) -> (22.741, 216.8058) ccw
  line L109 (22.741, 216.8058) -> (-123.259, 216.8058)
  ellipse E2 centre (-123.259, 209.5755) end of major axis (-123.259, 216.8058) minor radius 7 (-123.259, 216.8058) -> (-130.259, 209.5755) ccw
  line L110 (-130.259, 209.5755) -> (-130.259, -39.3535)
  ellipse E3 centre (-123.259, -39.3535) end of major axis (-123.259, -46.5838) minor radius 7 (-130.259, -39.3535) -> (-123.259, -46.5838) ccw
  line L111 (-123.259, -46.5838) -> (-60.0369, -46.5838)
  line L112 (-60.0369, -46.5838) -> (-60.0369, -43.8903)
  line L113 (-55, 10) -> (-55, 27.1913)
  line L114 (-63.1164, 198.8989) -> (-63.1164, 200.1093)
  line L115 (-63.1164, 200.1093) -> (-65.0274, 200.1093)
  line L116 (-65.0274, 200.1093) -> (-65.0274, 200.872)
  line L117 (-65.0274, 200.872) -> (-62.274, 200.8764)
  line L118 (-62.274, 200.8764) -> (-62.274, 198.4644)
  spline S0 degree 3 poles (-62.274, 198.4644) (-62.4834, 198.3077) (-62.8901, 198.0035) (-63.356, 197.8018) (-63.582, 197.704) knots 0 0 0 0 0.078157 0.151758 0.151758 0.151758 0.151758
  spline S1 degree 3 poles (-63.582, 197.704) (-63.8076, 197.6296) (-64.2571, 197.4815) (-64.7299, 197.4598) (-64.9653, 197.449) knots 0 0 0 0 0.070908 0.141252 0.141252 0.141252 0.141252
  spline S2 degree 3 poles (-64.9653, 197.449) (-65.2744, 197.4647) (-65.8798, 197.4952) (-66.4342, 197.7396) (-66.7056, 197.8592) knots 0 0 0 0 0.091966 0.180141 0.180141 0.180141 0.180141
  spline S3 degree 3 poles (-66.7056, 197.8592) (-66.9503, 198.0107) (-67.4379, 198.3127) (-67.7378, 198.8016) (-67.8872, 199.0452) knots 0 0 0 0 0.085037 0.169503 0.169503 0.169503 0.169503
  spline S4 degree 3 poles (-67.8872, 199.0452) (-68.0036, 199.3151) (-68.2421, 199.8684) (-68.2713, 200.4705) (-68.2863, 200.7789) knots 0 0 0 0 0.087419 0.179189 0.179189 0.179189 0.179189
  spline S5 degree 3 poles (-68.2863, 200.7789) (-68.2704, 201.0885) (-68.239, 201.7016) (-68.0052, 202.2692) (-67.8895, 202.5502) knots 0 0 0 0 0.09226 0.182704 0.182704 0.182704 0.182704
  spline S6 degree 3 poles (-67.8895, 202.5502) (-67.7454, 202.8052) (-67.4631, 203.3049) (-66.9829, 203.6183) (-66.7477, 203.7717) knots 0 0 0 0 0.086466 0.169395 0.169395 0.169395 0.169395
  spline S7 degree 3 poles (-66.7477, 203.7717) (-66.4845, 203.888) (-65.9383, 204.1295) (-65.3412, 204.1567) (-65.0319, 204.1707) knots 0 0 0 0 0.085548 0.177538 0.177538 0.177538 0.177538
  spline S8 degree 3 poles (-65.0319, 204.1707) (-64.8061, 204.1627) (-64.3702, 204.147) (-63.9566, 204.009) (-63.7571, 203.9424) knots 0 0 0 0 0.067359 0.130098 0.130098 0.130098 0.130098
  spline S9 degree 3 poles (-63.7571, 203.9424) (-63.58, 203.862) (-63.2405, 203.7078) (-62.9856, 203.4361) (-62.8637, 203.3061) knots 0 0 0 0 0.057702 0.110632 0.110632 0.110632 0.110632
  spline S10 degree 3 poles (-62.8637, 203.3061) (-62.7607, 203.1533) (-62.5397, 202.8254) (-62.4301, 202.445) (-62.3716, 202.242) knots 0 0 0 0 0.054958 0.117884 0.117884 0.117884 0.117884
  line L119 (-62.3716, 202.242) -> (-63.1475, 202.0292)
  spline S11 degree 3 poles (-63.1475, 202.0292) (-63.1952, 202.1803) (-63.2823, 202.4566) (-63.4397, 202.6995) (-63.5111, 202.8096) knots 0 0 0 0 0.047276 0.086437 0.086437 0.086437 0.086437
  spline S12 degree 3 poles (-63.5111, 202.8096) (-63.5945, 202.9008) (-63.7708, 203.0935) (-64.0072, 203.2052) (-64.1318, 203.264) knots 0 0 0 0 0.036726 0.077589 0.077589 0.077589 0.077589
  spline S13 degree 3 poles (-64.1318, 203.264) (-64.2723, 203.3138) (-64.562, 203.4164) (-64.8692, 203.4285) (-65.0274, 203.4347) knots 0 0 0 0 0.044449 0.091641 0.091641 0.091641 0.091641
  spline S14 degree 3 poles (-65.0274, 203.4347) (-65.2124, 203.4292) (-65.5614, 203.4188) (-65.8919, 203.3075) (-66.0472, 203.2552) knots 0 0 0 0 0.055163 0.104053 0.104053 0.104053 0.104053
  spline S15 degree 3 poles (-66.0472, 203.2552) (-66.1815, 203.1929) (-66.439, 203.0735) (-66.6434, 202.877) (-66.7411, 202.7829) knots 0 0 0 0 0.044061 0.084453 0.084453 0.084453 0.084453
  spline S16 degree 3 poles (-66.7411, 202.7829) (-66.8239, 202.6836) (-66.988, 202.4867) (-67.0971, 202.2549) (-67.1512, 202.14) knots 0 0 0 0 0.038631 0.076535 0.076535 0.076535 0.076535
  spline S17 degree 3 poles (-67.1512, 202.14) (-67.2236, 201.9325) (-67.3714, 201.509) (-67.39, 201.0607) (-67.3995, 200.8321) knots 0 0 0 0 0.06555 0.133782 0.133782 0.133782 0.133782
  spline S18 degree 3 poles (-67.3995, 200.8321) (-67.3911, 200.5625) (-67.3753, 200.0597) (-67.1874, 199.5938) (-67.1002, 199.3778) knots 0 0 0 0 0.080159 0.149513 0.149513 0.149513 0.149513
  spline S19 degree 3 poles (-67.1002, 199.3778) (-66.9899, 199.1956) (-66.7709, 198.8342) (-66.4087, 198.6166) (-66.229, 198.5087) knots 0 0 0 0 0.06285 0.12472 0.12472 0.12472 0.12472
  spline S20 degree 3 poles (-66.229, 198.5087) (-66.0352, 198.426) (-65.6469, 198.2601) (-65.2253, 198.2367) (-65.0141, 198.225) knots 0 0 0 0 0.062693 0.125611 0.125611 0.125611 0.125611
  spline S21 degree 3 poles (-65.0141, 198.225) (-64.8284, 198.2342) (-64.4544, 198.2527) (-64.1012, 198.3773) (-63.9234, 198.44) knots 0 0 0 0 0.055462 0.111696 0.111696 0.111696 0.111696
  spline S22 degree 3 poles (-63.9234, 198.44) (-63.7635, 198.5072) (-63.4759, 198.6281) (-63.227, 198.8156) (-63.1164, 198.8989) knots 0 0 0 0 0.051788 0.093147 0.093147 0.093147 0.093147
  spline S23 degree 3 poles (-54.9382, 198.3003) (-54.9002, 198.2836) (-54.8136, 198.2455) (-54.7187, 198.2437) (-54.6656, 198.2427) knots 0 0 0 0 0.012364 0.028114 0.028114 0.028114 0.028114
  spline S24 degree 3 poles (-54.6656, 198.2427) (-54.6141, 198.2445) (-54.4969, 198.2487) (-54.3806, 198.2647) (-54.3153, 198.2737) knots 0 0 0 0 0.015427 0.035185 0.035185 0.035185 0.035185
  line L120 (-54.3153, 198.2737) -> (-54.2, 197.5688)
  spline S25 degree 3 poles (-54.2, 197.5688) (-54.3061, 197.5481) (-54.5053, 197.5093) (-54.7082, 197.5015) (-54.803, 197.4978) knots 0 0 0 0 0.032364 0.060796 0.060796 0.060796 0.060796
  spline S26 degree 3 poles (-54.803, 197.4978) (-54.9335, 197.5003) (-55.1673, 197.5048) (-55.3821, 197.5953) (-55.4769, 197.6353) knots 0 0 0 0 0.038727 0.069335 0.069335 0.069335 0.069335
  spline S27 degree 3 poles (-55.4769, 197.6353) (-55.5503, 197.6834) (-55.6922, 197.7765) (-55.7742, 197.9249) (-55.8139, 197.9966) knots 0 0 0 0 0.025865 0.050076 0.050076 0.050076 0.050076
  spline S28 degree 3 poles (-55.8139, 197.9966) (-55.842, 198.112) (-55.917, 198.4208) (-55.9136, 198.7393) (-55.9115, 198.9388) knots 0 0 0 0 0.035512 0.095031 0.095031 0.095031 0.095031
  line L121 (-55.9115, 198.9388) -> (-55.9115, 201.6479)
  line L122 (-55.9115, 201.6479) -> (-56.4967, 201.6479)
  line L123 (-56.4967, 201.6479) -> (-56.4967, 202.2686)
  line L124 (-56.4967, 202.2686) -> (-55.9115, 202.2686)
  line L125 (-55.9115, 202.2686) -> (-55.9115, 203.4347)
  line L126 (-55.9115, 203.4347) -> (-55.1178, 203.9136)
  line L127 (-55.1178, 203.9136) -> (-55.1178, 202.2686)
  line L128 (-55.1178, 202.2686) -> (-54.3153, 202.2686)
  line L129 (-54.3153, 202.2686) -> (-54.3153, 201.6479)
  line L130 (-54.3153, 201.6479) -> (-55.1178, 201.6479)
  line L131 (-55.1178, 201.6479) -> (-55.1178, 198.8945)
  spline S29 degree 3 poles (-55.1178, 198.8945) (-55.119, 198.8004) (-55.1208, 198.6523) (-55.0878, 198.5082) (-55.0757, 198.4555) knots 0 0 0 0 0.028064 0.044226 0.044226 0.044226 0.044226
  spline S30 degree 3 poles (-55.0757, 198.4555) (-55.0592, 198.4246) (-55.0259, 198.3618) (-54.9677, 198.321) (-54.9382, 198.3003) knots 0 0 0 0 0.010363 0.020994 0.020994 0.020994 0.020994
  line L132 (-47.6823, 204.0599) -> (-47.6823, 203.1421)
  line L133 (-47.6823, 203.1421) -> (-48.4804, 203.1421)
  line L134 (-48.4804, 203.1421) -> (-48.4804, 204.0599)
  line L135 (-48.4804, 204.0599) -> (-47.6823, 204.0599)
  spline S31 degree 3 poles (-45.3434, 188.1557) (-45.3053, 188.139) (-45.2188, 188.1009) (-45.1239, 188.0991) (-45.0707, 188.0981) knots 0 0 0 0 0.012364 0.028115 0.028115 0.028115 0.028115
  spline S32 degree 3 poles (-45.0707, 188.0981) (-45.0193, 188.0999) (-44.902, 188.1041) (-44.7858, 188.1201) (-44.7205, 188.1291) knots 0 0 0 0 0.015427 0.035184 0.035184 0.035184 0.035184
  line L136 (-44.7205, 188.1291) -> (-44.6052, 187.4241)
  spline S33 degree 3 poles (-44.6052, 187.4241) (-44.7113, 187.4035) (-44.9105, 187.3647) (-45.1133, 187.3569) (-45.2082, 187.3532) knots 0 0 0 0 0.032364 0.060796 0.060796 0.060796 0.060796
  spline S34 degree 3 poles (-45.2082, 187.3532) (-45.3387, 187.3557) (-45.5725, 187.3602) (-45.7873, 187.4507) (-45.8821, 187.4907) knots 0 0 0 0 0.038727 0.069335 0.069335 0.069335 0.069335
  spline S35 degree 3 poles (-45.8821, 187.4907) (-45.9554, 187.5388) (-46.0974, 187.6319) (-46.1794, 187.7803) (-46.2191, 187.852) knots 0 0 0 0 0.025865 0.050076 0.050076 0.050076 0.050076
  spline S36 degree 3 poles (-46.2191, 187.852) (-46.2471, 187.9674) (-46.3222, 188.2761) (-46.3188, 188.5947) (-46.3166, 188.7942) knots 0 0 0 0 0.035512 0.095031 0.095031 0.095031 0.095031
  line L137 (-46.3166, 188.7942) -> (-46.3166, 191.5033)
  line L138 (-46.3166, 191.5033) -> (-46.9019, 191.5033)
  line L139 (-46.9019, 191.5033) -> (-46.9019, 192.124)
  line L140 (-46.9019, 192.124) -> (-46.3166, 192.124)
  line L141 (-46.3166, 192.124) -> (-46.3166, 193.2901)
  line L142 (-46.3166, 193.2901) -> (-45.523, 193.769)
  line L143 (-45.523, 193.769) -> (-45.523, 192.124)
  line L144 (-45.523, 192.124) -> (-44.7205, 192.124)
  line L145 (-44.7205, 192.124) -> (-44.7205, 191.5033)
  line L146 (-44.7205, 191.5033) -> (-45.523, 191.5033)
  line L147 (-45.523, 191.5033) -> (-45.523, 188.7499)
  spline S37 degree 3 poles (-45.523, 188.7499) (-45.5242, 188.6558) (-45.526, 188.5076) (-45.4929, 188.3636) (-45.4809, 188.3109) knots 0 0 0 0 0.028064 0.044226 0.044226 0.044226 0.044226
  spline S38 degree 3 poles (-45.4809, 188.3109) (-45.4644, 188.2799) (-45.4311, 188.2172) (-45.3729, 188.1764) (-45.3434, 188.1557) knots 0 0 0 0 0.010363 0.020994 0.020994 0.020994 0.020994
  line L148 (-67.1956, 190.3017) -> (-67.1956, 187.4153)
  line L149 (-67.1956, 187.4153) -> (-68.0557, 187.4153)
  line L150 (-68.0557, 187.4153) -> (-68.0557, 193.9153)
  line L151 (-68.0557, 193.9153) -> (-65.1737, 193.9153)
  spline S39 degree 3 poles (-65.1737, 193.9153) (-64.917, 193.9133) (-64.4685, 193.9099) (-64.0369, 193.791) (-63.8525, 193.7401) knots 0 0 0 0 0.076609 0.133783 0.133783 0.133783 0.133783
  spline S40 degree 3 poles (-63.8525, 193.7401) (-63.7085, 193.6693) (-63.4151, 193.5248) (-63.226, 193.2577) (-63.1297, 193.1216) knots 0 0 0 0 0.047344 0.096479 0.096479 0.096479 0.096479
  spline S41 degree 3 poles (-63.1297, 193.1216) (-63.0509, 192.9692) (-62.8917, 192.6617) (-62.8702, 192.3161) (-62.8593, 192.1417) knots 0 0 0 0 0.050884 0.102649 0.102649 0.102649 0.102649
  spline S42 degree 3 poles (-62.8593, 192.1417) (-62.8767, 191.9216) (-62.911, 191.4883) (-63.1765, 191.1447) (-63.3071, 190.9756) knots 0 0 0 0 0.064712 0.127351 0.127351 0.127351 0.127351
  spline S43 degree 3 poles (-63.3071, 190.9756) (-63.4898, 190.8304) (-63.8954, 190.5079) (-64.4084, 190.4206) (-64.6905, 190.3726) knots 0 0 0 0 0.068929 0.153084 0.153084 0.153084 0.153084
  spline S44 degree 3 poles (-64.6905, 190.3726) (-64.588, 190.322) (-64.4042, 190.2312) (-64.243, 190.1049) (-64.1717, 190.049) knots 0 0 0 0 0.034174 0.061288 0.061288 0.061288 0.061288
  spline S45 degree 3 poles (-64.1717, 190.049) (-64.0453, 189.9227) (-63.7798, 189.6574) (-63.5685, 189.347) (-63.4578, 189.1844) knots 0 0 0 0 0.053478 0.112342 0.112342 0.112342 0.112342
  line L152 (-63.4578, 189.1844) -> (-62.3272, 187.4153)
  line L153 (-62.3272, 187.4153) -> (-63.4091, 187.4153)
  line L154 (-63.4091, 187.4153) -> (-64.2692, 188.7676)
  spline S46 degree 3 poles (-64.2692, 188.7676) (-64.3816, 188.9413) (-64.5791, 189.2464) (-64.7964, 189.5377) (-64.89, 189.6632) knots 0 0 0 0 0.06204 0.108997 0.108997 0.108997 0.108997
  spline S47 degree 3 poles (-64.89, 189.6632) (-64.9633, 189.7549) (-65.0926, 189.9165) (-65.256, 190.043) (-65.3267, 190.0977) knots 0 0 0 0 0.035073 0.061797 0.061797 0.061797 0.061797
  spline S48 degree 3 poles (-65.3267, 190.0977) (-65.3903, 190.1357) (-65.514, 190.2097) (-65.652, 190.2507) (-65.7191, 190.2707) knots 0 0 0 0 0.022121 0.04303 0.04303 0.04303 0.04303
  spline S49 degree 3 poles (-65.7191, 190.2707) (-65.7833, 190.2796) (-65.942, 190.3018) (-66.1024, 190.3018) (-66.198, 190.3017) knots 0 0 0 0 0.019427 0.048036 0.048036 0.048036 0.048036
  line L155 (-66.198, 190.3017) -> (-67.1956, 190.3017)
  spline S50 degree 3 poles (-54.5192, 187.3089) (-54.7824, 187.3382) (-55.3103, 187.3972) (-55.6546, 187.8019) (-55.8272, 188.005) knots 0 0 0 0 0.076386 0.153256 0.153256 0.153256 0.153256
  line L156 (-55.8272, 188.005) -> (-55.8272, 187.4153)
  line L157 (-55.8272, 187.4153) -> (-56.5677, 187.4153)
  line L158 (-56.5677, 187.4153) -> (-56.5677, 193.9153)
  line L159 (-56.5677, 193.9153) -> (-55.7696, 193.9153)
  line L160 (-55.7696, 193.9153) -> (-55.7696, 191.5964)
  spline S51 degree 3 poles (-55.7696, 191.5964) (-55.5907, 191.7813) (-55.2364, 192.1477) (-54.7301, 192.203) (-54.4793, 192.2304) knots 0 0 0 0 0.074638 0.14787 0.14787 0.14787 0.14787
  spline S52 degree 3 poles (-54.4793, 192.2304) (-54.3368, 192.2233) (-54.0532, 192.2091) (-53.7885, 192.1064) (-53.6569, 192.0553) knots 0 0 0 0 0.042514 0.084577 0.084577 0.084577 0.084577
  spline S53 degree 3 poles (-53.6569, 192.0553) (-53.5338, 191.9917) (-53.2911, 191.8663) (-53.1085, 191.6633) (-53.0184, 191.5631) knots 0 0 0 0 0.041157 0.081209 0.081209 0.081209 0.081209
  spline S54 degree 3 poles (-53.0184, 191.5631) (-52.9386, 191.4493) (-52.7726, 191.2126) (-52.6761, 190.9399) (-52.626, 190.7983) knots 0 0 0 0 0.041496 0.086317 0.086317 0.086317 0.086317